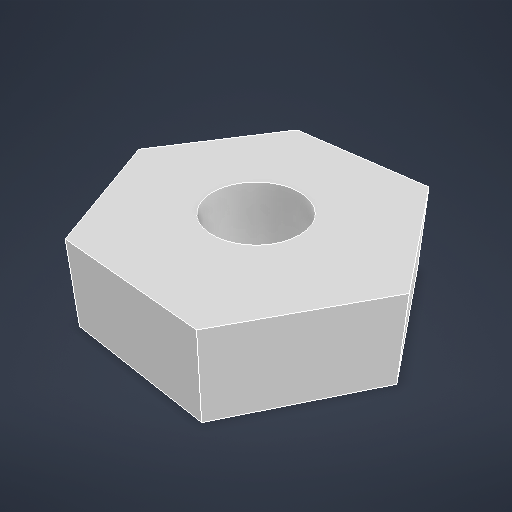
# Autodesk Inventor part: Front_Wheel_Support_Test
Saved by Autodesk Inventor 2025 (Build 290162000, 162)
## iProperties
Created: 2024-06-30
Part Number: Front_Wheel_Support_Test
Material: Generic
Document SubType Name: Modeling
Designer: Garfieldcmix
Density: 1 g/cm^3
Appearance: Default
Author: Garfieldcmix
Autodesk Inventor part; units mm, degrees
ref_plane "YZ Plane" through (0, 0, 0) normal (1, 0, 0) x (0, 1, 0)
ref_plane "XZ Plane" through (0, 0, 0) normal (0, 1, 0) x (-1, 0, 0)
ref_plane "XY Plane" through (0, 0, 0) normal (0, 0, 1) x (1, 0, 0)
sketch "Sketch1" plane through (0, 0, 0) normal (0, 1, 0) x (-1, 0, 0)
  circle A0 centre (0, 0) radius 2
  line L0 (-3.4641, -6) -> (3.4641, -6)
  line L1 (3.4641, -6) -> (6.9282, 0)
  line L2 (6.9282, 0) -> (3.4641, 6)
  line L3 (3.4641, 6) -> (-3.4641, 6)
  line L4 (-3.4641, 6) -> (-6.9282, 0)
  line L5 (-6.9282, 0) -> (-3.4641, -6)
  line L6 (0, 6) -> (0, -6) construction
  line L7 (-5.1962, 3) -> (5.1962, -3) construction
  line L8 (-5.1962, -3) -> (5.1962, 3) construction
  point P0 (0, 0)
  dimension "d0" = 4
  dimension "d1" = 12
  constraints: 18 end point, 7 midpoint, 5 equal length, 3 perpendicular, 2 coincident, 1 centre point, 1 vertical
  measures "d0" diameter of A0
  measures "d1" distance between parallel lines of L0 L3
extrude "Extrusion1" add sketch "Sketch1" along normal blind 4
offset faces "Size1" outward -0.18 faces at (-1.9935, 2.6667, -0.1609)
body "Solid1"
